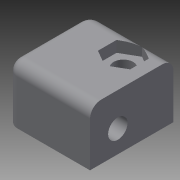
# Autodesk Inventor part: Z_endstop_regulator
Saved by Autodesk Inventor 2013 (Build 170138000, 138)
## iProperties
Created: 2014-02-06
Part Number: Z_endstop_regulator
Material: Ogólny
Document SubType Name: Modeling
Designer: Piotr
Density: 1 g/cm^3
Author: Piotr
Autodesk Inventor part; units mm, degrees
ref_plane "YZ Plane" through (0, 0, 0) normal (1, 0, 0) x (0, 1, 0)
ref_plane "XZ Plane" through (0, 0, 0) normal (0, 1, 0) x (-1, 0, 0)
ref_plane "XY Plane" through (0, 0, 0) normal (0, 0, 1) x (1, 0, 0)
sketch "Szkic1" plane through (0, 0, 0) normal (0, 0, 1) x (1, 0, 0)
  line L0 (-7.5, -7.5) -> (7.5, -7.5)
  line L1 (7.5, -7.5) -> (7.5, 7.5)
  line L2 (7.5, 7.5) -> (-7.5, 7.5)
  line L3 (-7.5, 7.5) -> (-7.5, -7.5)
  line L4 (-7.5, -7.5) -> (7.5, 7.5) construction
  line L5 (7.5, -7.5) -> (-7.5, 7.5) construction
  line L6 (7.5, 7.5) -> (2.5, 7.5) construction
  line L7 (2.5, 7.5) -> (2.5, 3.5) construction
  line L8 (2.5, 3.5) -> (7.5, 3.5) construction
  line L9 (7.5, 3.5) -> (7.5, 7.5) construction
  line L10 (2.5, 6.8486) -> (5.4, 5.1743)
  line L11 (5.4, 5.1743) -> (5.4, 1.8257)
  line L12 (5.4, 1.8257) -> (2.5, 0.1514)
  line L13 (2.5, 0.1514) -> (-0.4, 1.8257)
  line L14 (-0.4, 1.8257) -> (-0.4, 5.1743)
  line L15 (-0.4, 5.1743) -> (2.5, 6.8486)
  point P0 (0, 0)
  dimension "d0" = 15
  dimension "d1" = 15
  dimension "d4" = 5
  dimension "d5" = 4
  dimension "d8" = 5.8
  constraints: 32 end point, 4 parallel, 2 coincident, 2 horizontal, 2 midpoint, 2 perpendicular, 1 point on line, 13 other
  measures "d0" distance of L2.end L1.end
  measures "d1" distance of L1.end L0.end
  measures "d4" distance of L8.end L7.end
  measures "d5" distance of L7.end L6.end
  measures "d8" distance between parallel lines of L10 L13
extrude "Wyciągnięcie proste1" add sketch "Szkic1" along normal blind 10 contours L3 L2 L1 L0 | L10 L11 L12 L13 L14 L15
sketch "Szkic2" plane through (7.5, -7.5, 0) normal (1, 0, 0) x (0, 0, -1)
  line L0 (0, 0) -> (-4, 0) construction
  line L1 (-4, 0) -> (-4, 5) construction
  line L2 (-4, 5) -> (0, 5) construction
  line L3 (0, 5) -> (0, 0) construction
  point P0 (0, 7.5)
  dimension "d6" = 4
  dimension "d7" = 5
  constraints: 8 end point, 2 parallel, 1 coincident, 1 horizontal, 1 perpendicular
  measures "d6" distance of L1.end L2.end
  measures "d7" distance of L0.end L1.end
hole "Otwór1" at (2.5, 3.5, 0) direction (0, 0, 1) diameter 3.5 end through all
extrude "Wyciągnięcie proste2" cut sketch "Szkic1" along normal blind 3 contours L10 L11 L12 L13 L14 L15
hole "Otwór2" at (7.5, -2.5, 4) direction (-1, 0, 0) diameter 3.5 end through all
sketch "Szkic3" plane through (0, 0, 10) normal (0, 0, 1) x (1, 0, 0)
  circle A0 centre (2.5, 3.5) radius 1.75 projected
  line L0 (-0.4, 5.1743) -> (-0.4, 1.8257) projected
  line L1 (2.5, 6.8486) -> (-0.4, 5.1743) projected
  line L2 (2.5, 6.8486) -> (5.4, 5.1743) projected
  line L3 (5.4, 1.8257) -> (5.4, 5.1743) projected
  line L4 (2.5, 0.1514) -> (5.4, 1.8257) projected
  line L5 (2.5, 0.1514) -> (-0.4, 1.8257) projected
  point P0 (0, 0)
extrude "Wyciągnięcie proste3" cut sketch "Szkic3" against normal blind 2
fillet "Zaokrąglenie1" radius 2 5 edges at (-7.5, 7.5, 5) (-7.5, -7.5, 5) (-7.5, 0, 10) (0, 7.5, 10) (0, -7.5, 10)
sketch "Szkic4" plane through (0, 0, 3) normal (0, 0, -1) x (-1, 0, 0)
  circle A0 centre (-2.5, 3.5) radius 1.75 projected
  point P0 (0, 0)
extrude "Wyciągnięcie proste4" add sketch "Szkic4" against normal blind 0.5
